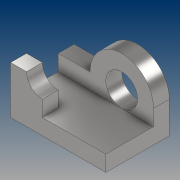
# Autodesk Inventor part: 7
Saved by Autodesk Inventor 2020.2 (Build 242310000, 310)
## iProperties
Created: 2020-09-17
Part Number: 7
Material: 鋼、碳鋼
Document SubType Name: Modeling
Designer: user
Density: 7.85 g/cm^3
Appearance: 半拋光
Mass: 285.396 g
Surface Area: 106.85 cm^2
Volume: 36.3562 cm^3
Author: user
Autodesk Inventor part; units mm, degrees
ref_plane "YZ Plane" through (0, 0, 0) normal (1, 0, 0) x (0, 1, 0)
ref_plane "XZ Plane" through (0, 0, 0) normal (0, 1, 0) x (-1, 0, 0)
ref_plane "XY Plane" through (0, 0, 0) normal (0, 0, 1) x (1, 0, 0)
sketch "草圖1" plane through (0, 0, 0) normal (0, 1, 0) x (-1, 0, 0)
  line L0 (30, 20) -> (-30, 20)
  line L1 (-30, 20) -> (-30, -20)
  line L2 (-30, -20) -> (30, -20)
  line L3 (30, -20) -> (30, 20)
  line L4 (30, 20) -> (-30, -20) construction
  line L5 (-30, 20) -> (30, -20) construction
  point P0 (0, 0)
  dimension "d0" = 60
  dimension "d1" = 40
  constraints: 12 end point, 2 midpoint, 2 parallel, 1 horizontal, 1 perpendicular
  measures "d0" distance of L0.start L0.end
  measures "d1" distance of L0.end L1.end
extrude "擠出1" add sketch "草圖1" along normal blind 10
sketch "草圖2" plane through (-30, 0, 20) normal (0, 0, 1) x (1, 0, 0)
  line L0 (0, 0) -> (0, 10) projected
  line L1 (0, 10) -> (60, 10) projected
  line L2 (60, 10) -> (60, 0) projected
  line L3 (60, 0) -> (0, 0) projected
  line L4 (60, 10) -> (0, 10) projected
  line L5 (0, 10) -> (0, 30)
  line L6 (0, 30) -> (10, 30)
  arc A0 (10, 30) -> (20, 20) centre (20, 30) ccw
  line L7 (20, 20) -> (20, 10)
  line L8 (0, 10) -> (60, 10) projected
  point P0 (30, 0)
  dimension "d4" = 20
  dimension "d5" = 30
  dimension "d6" = 10
  dimension "d7" = 10
  constraints: 6 end point, 2 point on circle, 2 point on line, 2 vertical, 1 centre point, 1 perpendicular
  measures "d4" distance between parallel lines of L7 L5
  measures "d5" distance between parallel lines of L3 L6
  measures "d6" distance of L7.start L7.end
  measures "d7" distance of L5.end L6.end
extrude "擠出2" add sketch "草圖2" against normal blind 10 contours L5 L6 A0 L7 L1
sketch "草圖3" plane through (30, 0, -20) normal (0, 0, -1) x (-1, 0, 0)
  line L0 (60, 10) -> (60, 0) projected
  line L1 (60, 0) -> (0, 0) projected
  line L2 (0, 0) -> (0, 10) projected
  line L3 (0, 10) -> (60, 10) projected
  line L4 (60, 10) -> (60, 20)
  line L5 (60, 20) -> (40, 20)
  line L6 (0, 10) -> (0, 20)
  arc A0 (40, 20) -> (0, 20) centre (20, 20) ccw
  point P0 (30, 0)
  dimension "d10" = 20
  dimension "d11" = 20
  constraints: 6 end point, 2 point on circle, 2 vertical, 1 centre point, 1 perpendicular, 1 point on line, 1 tangent
  measures "d10" distance between parallel lines of L1 L5
  measures "d11" distance from line of L6 A0.centre
extrude "擠出3" add sketch "草圖3" against normal blind 10 contours L3 L6 A0 L5 L4
sketch "草圖4" plane through (30, 0, -10) normal (0, 0, 1) x (1, 0, 0)
  arc A0 (0, 20) -> (-40, 20) centre (-20, 20) ccw projected
  point P0 (-30, 0)
  constraints: 1 coincident
hole "孔1" at (10, 20, -10) direction (0, 0, -1) diameter 20 end through all
